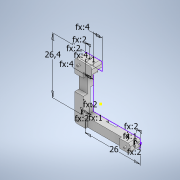
# Autodesk Inventor part: DisplayUnterlage
Saved by Autodesk Inventor 2022.2 (Build 262287010, 287A)
## iProperties
Created: 2022-02-23
Part Number: DisplayUnterlage
Material: Generisch
Document SubType Name: Modeling
Designer: hpcwoess
Density: 1 g/cm^3
Appearance: Vorgabe
Author: hpcwoess
Autodesk Inventor part; units mm, degrees
ref_plane "YZ Plane" through (0, 0, 0) normal (1, 0, 0) x (0, 1, 0)
ref_plane "XZ Plane" through (0, 0, 0) normal (0, 1, 0) x (-1, 0, 0)
ref_plane "XY Plane" through (0, 0, 0) normal (0, 0, 1) x (1, 0, 0)
sketch "Skizze1" plane through (0, 0, 0) normal (0, 0, 1) x (1, 0, 0)
  line L0 (0.6661, 17.7191) -> (-7.3339, 17.7191)
  line L1 (-7.3339, 17.7191) -> (-7.3339, -8.6809)
  line L2 (-7.3339, -8.6809) -> (18.6661, -8.6809)
  line L3 (18.6661, -8.6809) -> (18.6661, -4.6809)
  line L4 (18.6661, -4.6809) -> (-3.3339, -4.6809)
  line L5 (-3.3339, -4.6809) -> (-3.3339, 13.7191)
  line L6 (-3.3339, 13.7191) -> (0.6661, 13.7191)
  line L7 (0.6661, 13.7191) -> (0.6661, 17.7191)
  circle A0 centre (-5.3339, 15.7191) radius 0.5
  circle A1 centre (-5.3339, -6.6809) radius 0.5
  circle A2 centre (16.6661, -6.6809) radius 0.5
  point P0 (0, 0)
  point P1 (18.6661, -6.6809)
  point P2 (-1.3339, 13.7191)
  dimension "d0" = 26
  dimension "d1" = 26.4
  dimension "d2" = 4
  dimension "d3" = 4
  dimension "d4" = 4
  dimension "d5" = 4
  dimension "d6" = 1
  dimension "d7" = 1
  dimension "d8" = 1
  dimension "d9" = 2
  dimension "d10" = 2
  dimension "d11" = 2
  dimension "d12" = 2
  dimension "d13" = 2
  dimension "d14" = 2
  constraints: 16 end point, 7 perpendicular, 3 centre point, 2 midpoint, 1 horizontal
  measures "d0" distance from line of point (18.666, -6.681) L1
  measures "d1" distance between parallel lines of L0 L2
  measures "d2" distance between parallel lines of L4 L2
  measures "d3" distance between parallel lines of L5 L1
  measures "d4" distance from line of L0 point (-1.334, 13.719)
  measures "d5" distance between parallel lines of L7 L5
  measures "d6" diameter of A0
  measures "d7" diameter of A1
  measures "d8" diameter of A2
  measures "d9" distance from line of L1 A0.centre
  measures "d10" distance from line of L0 A0.centre
  measures "d11" distance from line of L2 A1.centre
  measures "d12" distance from line of L1 A1.centre
  measures "d13" distance from line of L2 A2.centre
  measures "d14" distance from line of L3 A2.centre
extrude "Extrusion1" add sketch "Skizze1" along normal blind 4.8 contours L7 L6 L5 L4 L3 L2 L1 L0 | A0 | A1 | A2
extrude "Extrusion2" add sketch "Skizze1" along normal blind 5.7 contours A0 | A1 | A2
chamfer "Fase1" distance 0.2 angle 45 1 edges at (-5.8339, 15.7191, 5.7)
chamfer "Fase2" distance 0.2 angle 45 2 edges at (-5.8339, -6.6809, 5.7) (16.1661, -6.6809, 5.7)
sketch "Skizze2" plane through (-7.3339, -8.6809, 0) normal (0, -1, 0) x (1, 0, 0)
  line L0 (5, 5.5045) -> (21, 5.5045)
  line L1 (21, 5.5045) -> (21, 3.8)
  line L2 (21, 3.8) -> (5, 3.8)
  line L3 (5, 3.8) -> (5, 5.5045)
  line L4 (0, 0) -> (0, 4.8) projected
  line L5 (26, 0) -> (26, 4.8) projected
  line L6 (0, 4.8) -> (26, 4.8) projected
  line L7 (11.1841, -1.1388) -> (15.6513, -1.1388)
  line L8 (15.6513, -1.1388) -> (15.6513, 1.113)
  line L9 (15.6513, 1.113) -> (11.1841, 1.113)
  line L10 (11.1841, 1.113) -> (11.1841, -1.1388)
  point P0 (7.3339, 0)
  point P1 (21, 4.6522)
  dimension "d25" = 16
  dimension "d26" = 26
  dimension "d27" = 5
  dimension "d28" = 1
  constraints: 16 end point, 4 parallel, 2 horizontal, 2 perpendicular, 1 midpoint
  measures "d25" distance of L1.end L2.end
  measures "d26" distance between parallel lines of L4 L5
  measures "d27" distance from line of point (21, 4.652) L5
  measures "d28" distance between parallel lines of L6 L2
extrude "Extrusion3" cut sketch "Skizze2" against normal blind 5.7
sketch "Skizze3" plane through (-7.3339, -8.6809, 0) normal (-1, 0, 0) x (0, 0, 1)
  line L0 (6.3376, 19.9761) -> (2.8, 19.9761)
  line L1 (2.8, 19.9761) -> (2.8, 12.567)
  line L2 (2.8, 12.567) -> (6.3376, 12.567)
  line L3 (6.3376, 12.567) -> (6.3376, 19.9761)
  line L4 (-2.0066, 6.6289) -> (1.5, 6.6289)
  line L5 (1.5, 6.6289) -> (1.5, 14.728)
  line L6 (1.5, 14.728) -> (-2.0066, 14.728)
  line L7 (-2.0066, 14.728) -> (-2.0066, 6.6289)
  line L8 (4.8, 26.4) -> (4.8, 0) projected
  line L9 (0, 26.4) -> (0, 0) projected
  point P0 (0, 8.6809)
  dimension "d33" = 2
  dimension "d34" = 1.5
  constraints: 16 end point, 4 parallel, 2 horizontal, 2 perpendicular
  measures "d33" distance between parallel lines of L8 L1
  measures "d34" distance between parallel lines of L9 L5
extrude "Extrusion4" cut sketch "Skizze3" against normal blind 5.7
fillet "Rundung1" radius 1 1 edges at (18.6661, -8.6809, 2.4)
fillet "Rundung2" radius 1 5 edges at (0.6661, 13.7191, 2.4) (18.6661, -4.6809, 2.4) (0.6661, 17.7191, 2.4) (-7.3339, -8.6809, 2.4) (-7.3339, 17.7191, 2.4)
sketch "Skizze4" plane through (-7.3339, -2.052, 1.5) normal (-1, 0, 0) x (0, 0, 1)
  line L0 (-1.5, 8.0991) -> (-1.5, 15.7711) projected
  line L1 (-1.5, 14.5578) -> (0.4295, 14.5578)
  line L2 (0.4295, 14.5578) -> (0.4295, 17.4567)
  line L3 (0.4295, 17.4567) -> (-1.5, 17.4567)
  line L4 (-1.5, 17.4567) -> (-1.5, 14.5578)
  point P0 (-1.5, 2.052)
  point P1 (-1.5, 15.7711)
  constraints: 8 end point, 2 parallel, 1 horizontal, 1 perpendicular, 1 point on line
extrude "Extrusion5" cut sketch "Skizze4" against normal blind 10
equation "\"d3\" = d2"
equation "\"d4\" = d3"
equation "\"d5\" = d4"
equation "\"d7\" = d6"
equation "\"d8\" = d6"
equation "\"d9\" = 0.5 * d4"
equation "\"d10\" = d9"
equation "\"d11\" = d10"
equation "\"d12\" = d10"
equation "\"d13\" = d11"
equation "\"d14\" = d13"
equation "\"d27\" = -0.5 * d25 + 0.5 * d26"
